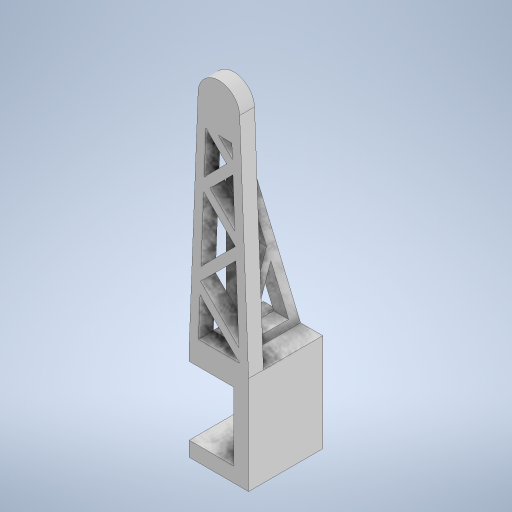
# Autodesk Inventor part: 전체 형상
Saved by Autodesk Inventor 2023 (Build 270158000, 158)
## iProperties
Created: 2022-11-11
Part Number: 전체 형상
Material: 일반
Document SubType Name: Modeling
Designer: hyunsu
Density: 1 g/cm^3
Appearance: 기본값
Author: hyunsu
Autodesk Inventor part; units mm, degrees
ref_plane "YZ Plane" through (0, 0, 0) normal (1, 0, 0) x (0, 1, 0)
ref_plane "XZ Plane" through (0, 0, 0) normal (0, 1, 0) x (-1, 0, 0)
sketch "스케치1" plane through (0, 0, 0) normal (0, 0, 1) x (1, 0, 0)
  line L0 (-5, -33) -> (5, -33)
  line L1 (5, -33) -> (5, 33)
  line L2 (5, 33) -> (-5, 33)
  line L3 (-5, 33) -> (-5, -33)
  line L4 (-5, -33) -> (5, 33) construction
  line L5 (5, -33) -> (-5, 33) construction
  line L6 (-5, 33) -> (-35, 33)
  line L7 (-35, 33) -> (-35, 23)
  line L8 (-35, 23) -> (-5, 23)
  line L9 (-5, 23) -> (-5, 33)
  line L10 (0, 0) -> (-11.0402, 0)
  line L11 (-5, -33) -> (-35, -33)
  line L12 (-35, -33) -> (-35, -23)
  line L13 (-35, -23) -> (-5, -23)
  point P0 (-5, 23)
  point P1 (-5, -23)
  dimension "d0" = 66
  dimension "d1" = 10
  dimension "d2" = 10
  dimension "d3" = 30
  constraints: 28 end point, 4 parallel, 3 horizontal, 3 symmetric about line, 2 midpoint, 2 perpendicular
  measures "d0" distance of L0.end L1.end
  measures "d1" distance of L1.end L2.end
  measures "d2" distance of L6.end L7.end
  measures "d3" distance of L2.end L6.end
extrude "돌출1" add sketch "스케치1" along normal mid plane 50
sketch "스케치2" plane through (0, 0, 25) normal (0, 0, 1) x (1, 0, 0)
  circle A0 centre (-15, 183) radius 14
  line L0 (-35, 33) -> (-35, 23) projected
  line L1 (-35, 33) -> (-28.9889, 183.5585)
  line L2 (5, 33) -> (-35, 33) projected
  line L3 (-15, 33) -> (-15, 183) construction
  line L4 (5, 33) -> (-1.0111, 183.5585)
  point P0 (0, 0)
  dimension "d6" = 28
  dimension "d17" = 6
  dimension "d7" = 150
  constraints: 6 end point, 1 coincident, 1 midpoint, 1 symmetric about line, 1 vertical, 4 other
  measures "d7" distance of L3.start L3.end
extrude "돌출2" add sketch "스케치2" against normal blind 10
ref_plane "작업 평면1" through (-15, 23, -25) normal (-1, 0, 0) x (0, 0, 1)
sketch "스케치3" plane through (-15, 23, -25) normal (-1, 0, 0) x (0, 0, 1)
  line L0 (40, 160.5585) -> (40, 10) projected
  line L1 (0, 10) -> (40, 10) projected
  line L2 (40, 144.5585) -> (0, 10)
  line L3 (45.7513, 142.8488) -> (8.0431, 16)
  line L4 (8.0431, 16) -> (34, 16)
  line L5 (34, 16) -> (34, 160.5585)
  line L6 (34, 16) -> (20, 56.2226)
  line L7 (34, 34.2526) -> (22.9265, 66.0672)
  point P0 (25, -23)
  point P1 (34, 103.318)
  point P2 (34, 124.3747)
  point P3 (40, 123.5018)
  dimension "d10" = 16
  dimension "d11" = 6
  dimension "d12" = 6
  constraints: 12 end point, 4 point on line, 1 parallel, 2 other
  measures "d10" distance of L0.start L2.start
  measures "d11" distance between parallel lines of L2 L3
  measures "d12" distance between parallel lines of L6 L7
extrude "돌출3" add sketch "스케치3" along normal mid plane 10 contours L0 L3 L5 L2 | L0 L1 L2 L5 L3 | L7 L5 L6 L3
sketch "스케치4" plane through (0, 0, 25) normal (0, 0, 1) x (1, 0, 0)
  line L0 (-35, 33) -> (-28.9889, 183.5585) projected
  line L1 (5, 33) -> (-1.0111, 183.5585) projected
  line L2 (-35, 33) -> (5, 33)
  arc A0 (-1.0111, 183.5585) -> (-28.9889, 183.5585) centre (-15, 183) ccw projected
  line L3 (-7.0064, 183.3192) -> (-1.2443, 39)
  line L4 (-1.2443, 39) -> (-28.7557, 39)
  line L5 (-28.7557, 39) -> (-22.9936, 183.3192)
  arc A1 (-7.0064, 183.3192) -> (-22.9936, 183.3192) centre (-15, 183) ccw
  line L6 (-1.2443, 39) -> (-27.6994, 65.4551)
  line L7 (-1.5972, 47.8382) -> (-27.3737, 73.6146)
  line L8 (-27.3737, 73.6146) -> (-3.5765, 97.4118)
  line L9 (-3.9022, 105.5713) -> (-27.0208, 82.4528)
  line L10 (-3.9022, 105.5713) -> (-25.2456, 126.9147)
  line L11 (-25.2456, 126.9147) -> (-5.5411, 146.6192)
  line L12 (-5.5411, 146.6192) -> (-23.7326, 164.8107)
  line L13 (-23.7326, 164.8107) -> (-6.2674, 164.8107)
  line L14 (-21.003, 131.1573) -> (-4.2551, 114.4095)
  line L15 (-15.2473, 164.8107) -> (-5.894, 155.4574)
  line L16 (-24.8927, 135.7528) -> (-9.7837, 150.8618)
  point P0 (0, 0)
  point P1 (-5.2153, 138.4597)
  dimension "d15" = 6
  dimension "d16" = 45
  dimension "d17" = 6
  dimension "d18" = 90
  dimension "d19" = 6
  dimension "d23" = 6
  constraints: 28 end point, 9 point on line, 3 parallel, 3 perpendicular, 2 horizontal, 2 point on circle, 1 centre point, 14 other
  measures "d16" angle of L4 L6
  measures "d17" distance between parallel lines of L6 L7
  measures "d18" angle of L7 L8
  measures "d19" distance between parallel lines of L8 L9
  measures "d23" distance between parallel lines of L16 L11
extrude "돌출4" cut sketch "스케치4" against normal blind 10 contours L3 L15 L13 | L12 L16 L5 | L3 L14 L11 | L10 L9 L5 | L3 L7 L8 | L6 L4 L5
